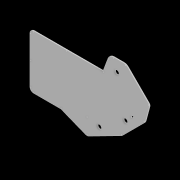
# Autodesk Inventor part: electronics-cover
Saved by Autodesk Inventor 2020 (Build 240168000, 168)
## iProperties
Created: 2020-02-02
Part Number: electronics-cover
Material: Generic
Document SubType Name: Modeling
Designer: valer
Density: 1 g/cm^3
Appearance: Default
Author: valer
Autodesk Inventor part; units mm, degrees
ref_plane "YZ Plane" through (0, 0, 0) normal (1, 0, 0) x (0, 1, 0)
ref_plane "XZ Plane" through (0, 0, 0) normal (0, 1, 0) x (-1, 0, 0)
ref_plane "XY Plane" through (0, 0, 0) normal (0, 0, 1) x (1, 0, 0)
sketch "Profile" plane through (0, 0, 0) normal (0, 0, 1) x (1, 0, 0)
  arc A0 (-133.951, 77.8406) -> (-145.3411, 66.4505) centre (-133.951, 66.4505) ccw
  line L0 (-133.951, 77.8406) -> (-53.1048, 77.8406)
  line L1 (-34.3215, 77.8406) -> (75.2802, 77.8406)
  line L2 (-53.1048, 77.8406) -> (-34.3215, 77.8406)
  arc A1 (75.2802, 77.8406) -> (76.5082, 78.6945) centre (75.2802, 79.1505) ccw
  line L3 (76.5082, 78.6945) -> (91.3749, 118.7338)
  arc A2 (108.0055, 130.2989) -> (91.3749, 118.7338) centre (108.0055, 112.5588) ccw
  line L4 (108.0055, 130.2989) -> (138.3634, 130.2989)
  arc A3 (150.9075, 125.103) -> (138.3634, 130.2989) centre (138.3634, 112.5588) ccw
  line L5 (150.9075, 125.103) -> (214.354, 61.6565)
  arc A4 (216.4802, 53.7213) -> (214.354, 61.6565) centre (208.545, 55.8476) ccw
  line L6 (216.4802, 53.7213) -> (205.0854, 11.1954)
  arc A5 (200.4939, 3.2427) -> (205.0854, 11.1954) centre (187.9498, 15.7868) ccw
  line L7 (200.4939, 3.2427) -> (135.4341, -61.8171)
  arc A6 (132.5618, -63.9063) -> (135.4341, -61.8171) centre (127.3801, -53.7631) ccw
  line L8 (132.5618, -63.9063) -> (33.0352, -114.7498)
  arc A7 (23.6561, -115.1951) -> (33.0352, -114.7498) centre (27.8535, -104.6066) ccw
  line L9 (23.6561, -115.1951) -> (-50.4135, -85.8326)
  arc A8 (-50.4135, -85.8326) -> (-51.6732, -85.5921) centre (-51.6732, -89.0102) ccw
  line L10 (-51.6732, -85.5921) -> (-133.951, -85.5921)
  arc A9 (-145.3411, -74.202) -> (-133.951, -85.5921) centre (-133.951, -74.202) ccw
  line L11 (-145.3411, -74.202) -> (-145.3411, 66.4505)
  circle A10 centre (-133.951, 75.3205) radius 1.27
  circle A11 centre (-142.8211, 66.4505) radius 1.27
  circle A12 centre (-34.3215, 75.3205) radius 1.27
  circle A13 centre (77.4668, 76.0061) radius 1.27
  circle A14 centre (93.7373, 117.8567) radius 1.27
  circle A15 centre (108.0055, 127.7789) radius 1.27
  circle A16 centre (144.1878, 126.6203) radius 1.27
  circle A17 centre (214.046, 57.3215) radius 1.27
  circle A18 centre (201.1307, 8.1768) radius 1.27
  circle A19 centre (132.5975, -60.9364) radius 1.27
  circle A20 centre (28.2741, -113.4667) radius 1.27
  circle A21 centre (-50.5593, -83.1775) radius 1.27
  circle A22 centre (-133.951, -83.072) radius 1.27
  circle A23 centre (-142.8211, -74.202) radius 1.27
  circle A24 centre (-142.8211, -3.8758) radius 1.27
  line L12 (28.2741, -113.4667) -> (28.2741, -66.8831) construction
  circle A25 centre (28.2741, -66.8831) radius 1.27
  point P0 (0, 0)
  dimension "d2" = 46.5836
  constraints: 26 centre point, 26 end point, 20 point on circle, 5 horizontal, 2 vertical, 1 coincident, 1 equal radius, 30 other
  measures "d2" distance of L12.start L12.end
extrude "BaseFeature" add sketch "Profile" along normal blind 2.54
sketch "BatteryMount" plane through (0, 0, 2.54) normal (0, 0, 1) x (1, 0, 0)
  circle A0 centre (118.5889, 95.5009) radius 6.35
  circle A1 centre (118.5889, 95.5009) radius 6.35
  arc A2 (102.7139, 117.5989) -> (99.5389, 114.4239) centre (102.7139, 114.4239) ccw
  line L0 (99.5389, 114.4239) -> (99.5389, 76.5779)
  arc A3 (99.5389, 76.5779) -> (102.7139, 73.4029) centre (102.7139, 76.5779) ccw
  line L1 (102.7139, 73.4029) -> (134.4639, 73.4029)
  arc A4 (134.4639, 73.4029) -> (137.6389, 76.5779) centre (134.4639, 76.5779) ccw
  line L2 (137.6389, 76.5779) -> (137.6389, 114.4239)
  arc A5 (137.6389, 114.4239) -> (134.4639, 117.5989) centre (134.4639, 114.4239) ccw
  line L3 (134.4639, 117.5989) -> (102.7139, 117.5989)
  line L4 (138.3634, 130.2989) -> (108.0055, 130.2989) projected
  point P0 (0, 0)
  dimension "d3" = 37.846
  dimension "d4" = 31.75
  dimension "d5" = 3.175
  dimension "d6" = 12.7
  dimension "d7" = 22.098
  dimension "d8" = 19.05
  dimension "d9" = 12.7
  dimension "d10" = 8.4667
  constraints: 8 end point, 8 point on circle, 6 centre point, 6 tangent, 3 equal radius, 3 parallel, 3 perpendicular, 2 coincident
  measures "d3" distance of L2.start L2.end
  measures "d4" distance of L1.start L1.end
  measures "d5" radius of A5
  measures "d6" diameter of A0
  measures "d7" distance from line of L3 point (118.589, 95.501)
  measures "d8" distance from line of L0 point (118.589, 95.501)
  measures "d9" distance between parallel lines of L4 L3
  measures "d10" distance from line of L4.end L0
extrude "BatteryMountFeature" cut sketch "BatteryMount" against normal through all contours A0
sketch "Outputs" plane through (0, 0, 2.54) normal (0, 0, 1) x (1, 0, 0)
  circle A0 centre (65.5047, -73.9186) radius 6.35
  circle A1 centre (144.5693, -18.557) radius 6.35
  line L0 (135.4341, -61.8171) -> (200.4939, 3.2427) projected
  line L1 (33.0352, -114.7498) -> (132.5618, -63.9063) construction
  line L2 (144.5693, -18.557) -> (65.5047, -73.9186) construction
  point P0 (0, 0)
  dimension "d13" = 12.7
  dimension "d14" = 24.13
  dimension "d15" = 21.59
  dimension "d16" = 10
  dimension "d17" = 96.52
  constraints: 2 centre point, 2 end point, 1 equal radius
  measures "d13" diameter of A0
  measures "d14" distance from line of L0 L2.start
  measures "d15" distance from line of L1 L2.end
  measures "d16" angle of L0 L2
  measures "d17" distance of L2.start L2.end
extrude "OutputHolesFeature" cut sketch "Outputs" against normal through all
sketch "USB-CInput" plane through (0, 0, 2.54) normal (0, 0, 1) x (1, 0, 0)
  circle A0 centre (162.5298, -0.5965) radius 1.5875
  circle A1 centre (167.0199, 3.8937) radius 1.5875
  line L0 (162.5298, -0.5965) -> (167.0199, 3.8937) construction
  line L1 (135.4341, -61.8171) -> (200.4939, 3.2427) construction
  circle A2 centre (144.5693, -18.557) radius 6.35 construction
  line L2 (162.5298, -0.5965) -> (144.5693, -18.557) construction
  line L3 (161.4072, 0.5261) -> (165.8974, 5.0162)
  line L4 (168.1424, 2.7711) -> (163.6523, -1.719)
  point P0 (0, 0)
  dimension "d20" = 3.175
  dimension "d21" = 25.4
  dimension "d22" = 6.35
  constraints: 8 end point, 4 point on circle, 4 tangent, 2 centre point, 1 collinear, 1 equal radius, 1 parallel
  measures "d20" diameter of A1
  measures "d21" distance of L0.start L2.end
  measures "d22" distance of L0.start L0.end
extrude "USB-CInputFeature" cut sketch "USB-CInput" against normal through all
body "Solid1"
